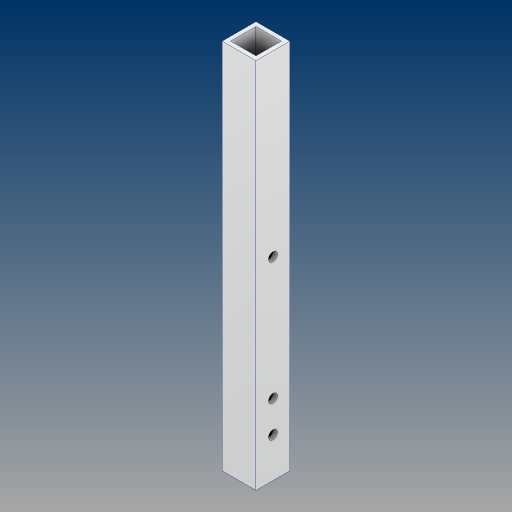
# Autodesk Inventor part: STRU_023_Kenji_11in
Saved by Autodesk Inventor 2024.3 (Build 283343000, 343)
## iProperties
Created: 2024-08-02
Part Number: STRU_023_Kenji_11in
Material: Aluminum 6061
Document SubType Name: Modeling
Designer: Bryan
Density: 2.7 g/cm^3
Appearance: Aluminum - Flat
Author: Bryan
Autodesk Inventor part; units mm, degrees
ref_plane "YZ Plane" through (0, 0, 0) normal (1, 0, 0) x (0, 1, 0)
ref_plane "XZ Plane" through (0, 0, 0) normal (0, 1, 0) x (-1, 0, 0)
ref_plane "XY Plane" through (0, 0, 0) normal (0, 0, 1) x (1, 0, 0)
sketch "Sketch1" plane through (0, 0, 0) normal (0, 1, 0) x (-1, 0, 0)
  line L0 (-12.7, -12.7) -> (12.7, -12.7)
  line L1 (12.7, -12.7) -> (12.7, 12.7)
  line L2 (12.7, 12.7) -> (-12.7, 12.7)
  line L3 (-12.7, 12.7) -> (-12.7, -12.7)
  line L4 (-12.7, -12.7) -> (12.7, 12.7) construction
  line L5 (12.7, -12.7) -> (-12.7, 12.7) construction
  line L6 (-9.525, 9.525) -> (9.525, 9.525)
  line L7 (9.525, 9.525) -> (9.525, -9.525)
  line L8 (9.525, -9.525) -> (-9.525, -9.525)
  line L9 (-9.525, -9.525) -> (-9.525, 9.525)
  point P0 (0, 0)
  dimension "d0" = 25.4
  dimension "d1" = 25.4
  dimension "d2" = 3.175
  constraints: 20 end point, 4 parallel, 2 midpoint, 2 perpendicular, 1 horizontal, 3 other
  measures "d0" distance of L2.end L1.end
  measures "d1" distance of L1.end L0.end
  measures "d2" distance between parallel lines of L2 L6
extrude "Extrusion1" add sketch "Sketch1" along normal blind 279.4
sketch "Sketch2" plane through (-12.7, 0, -12.7) normal (-1, 0, 0) x (0, 0, 1)
  line L0 (22.225, 279.4) -> (3.175, 279.4) projected
  line L1 (12.7, 279.4) -> (12.7, 145.6182) construction
  line L2 (12.7, 0) -> (12.7, 29.845) construction
  circle A0 centre (12.7, 145.6182) radius 3.2512
  circle A1 centre (12.7, 29.845) radius 3.2512
  line L3 (12.7, 0) -> (12.7, 53.467) construction
  circle A2 centre (12.7, 53.467) radius 3.2512
  line L4 (0, 0) -> (25.4, 0) construction
  dimension "d5" = 6.5024
  dimension "d6" = 133.7818
  dimension "d7" = 6.5024
  dimension "d8" = 29.845
  dimension "d11" = 53.467
  dimension "d12" = 6.5024
  constraints: 6 end point, 3 centre point, 3 coincident, 3 vertical, 2 midpoint, 1 collinear
  measures "d5" diameter of A0
  measures "d6" distance of L1.start L1.end
  measures "d7" diameter of A1
  measures "d8" distance of L2.start L2.end
  measures "d11" distance of L3.start L3.end
  measures "d12" diameter of A2
extrude "Extrusion2" cut sketch "Sketch2" against normal blind 25.4 contours A0 | A1
extrude "Extrusion3" cut sketch "Sketch2" against normal blind 25.4 contours A2
body "Solid1"
